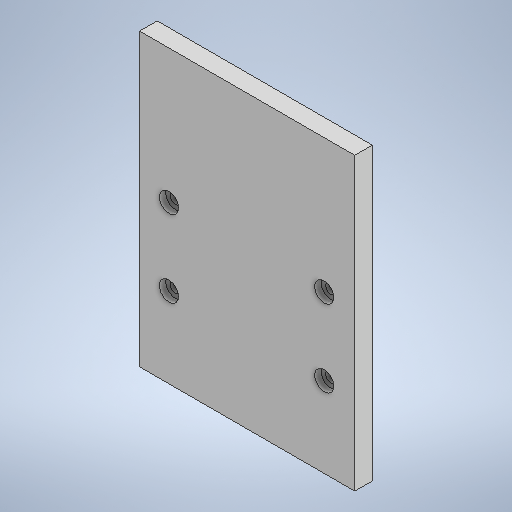
# Autodesk Inventor part: TES_ESP32-Case
Saved by Autodesk Inventor 2025 (Build 290162000, 162)
## iProperties
Created: 2025-08-28
Part Number: TES_ESP32-Case
Material: 常规
Document SubType Name: Modeling
Designer: user
Density: 1 g/cm^3
Appearance: 默认
Author: user
Autodesk Inventor part; units mm, degrees
ref_plane "YZ Plane" through (0, 0, 0) normal (1, 0, 0) x (0, 1, 0)
ref_plane "XZ Plane" through (0, 0, 0) normal (0, 1, 0) x (-1, 0, 0)
ref_plane "XY Plane" through (0, 0, 0) normal (0, 0, 1) x (1, 0, 0)
sketch "草图1" plane through (0, 0, 0) normal (0, 0, 1) x (1, 0, 0)
  line L0 (32.05, -44.65) -> (-32.05, -44.65)
  line L1 (-32.05, -44.65) -> (-32.05, 44.65)
  line L2 (-32.05, 44.65) -> (32.05, 44.65)
  line L3 (32.05, 44.65) -> (32.05, -44.65)
  line L4 (32.05, -44.65) -> (-32.05, 44.65) construction
  line L5 (-32.05, -44.65) -> (32.05, 44.65) construction
  line L6 (24.111, -19.563) -> (-24.389, -19.563) construction
  line L7 (-24.389, -19.563) -> (-24.389, 4.437) construction
  line L8 (-24.389, 4.437) -> (24.111, 4.437) construction
  line L9 (24.111, 4.437) -> (24.111, -19.563) construction
  line L10 (24.111, -19.563) -> (-24.389, 4.437) construction
  line L11 (-24.389, -19.563) -> (24.111, 4.437) construction
  circle A0 centre (-24.389, 4.437) radius 1.6
  circle A1 centre (-24.389, -19.563) radius 1.6
  circle A2 centre (24.111, 4.437) radius 1.6
  circle A3 centre (24.111, -19.563) radius 1.6
  line L12 (29.55, -43.15) -> (-4.45, -43.15)
  line L13 (-4.45, -43.15) -> (-4.45, -38.15)
  line L14 (-4.45, -38.15) -> (29.55, -38.15)
  line L15 (29.55, -38.15) -> (29.55, -43.15)
  line L16 (-19.55, -38.15) -> (-7.55, -38.15)
  line L17 (-7.55, -38.15) -> (-7.55, -33.65)
  line L18 (-7.55, -33.65) -> (-19.55, -33.65)
  line L19 (-19.55, -33.65) -> (-19.55, -38.15)
  line L20 (-20.05, -32.65) -> (-29.05, -32.65)
  line L21 (-29.05, -32.65) -> (-29.05, -28.15)
  line L22 (-29.05, -28.15) -> (-20.05, -28.15)
  line L23 (-20.05, -28.15) -> (-20.05, -32.65)
  line L24 (-12.05, 20.15) -> (-0.05, 20.15)
  line L25 (-0.05, 20.15) -> (-0.05, 24.65)
  line L26 (-0.05, 24.65) -> (-12.05, 24.65)
  line L27 (-12.05, 24.65) -> (-12.05, 20.15)
  point P0 (0, 0)
  point P1 (-0.139, -7.563)
  point P2 (-20.05, -30.4)
  dimension "d0" = 64.1
  dimension "d1" = 89.3
  dimension "d2" = 48.5
  dimension "d3" = 24
  dimension "d4" = 52.213
  dimension "d5" = 37.087
  dimension "d6" = 32.189
  dimension "d7" = 31.911
  dimension "d8" = 3.2
  dimension "d9" = 3.2
  dimension "d10" = 3.2
  dimension "d11" = 3.2
  dimension "d16" = 6.5
  dimension "d20" = 24.5
  dimension "d21" = 36.5
  dimension "d22" = 12.5
  dimension "d23" = 11
  dimension "d24" = 6.5
  dimension "d25" = 2.5
  dimension "d26" = 1.5
  dimension "d27" = 12
  dimension "d28" = 12
  dimension "d29" = 3
  dimension "d30" = 16.5
  dimension "d31" = 32
  dimension "d32" = 20
  dimension "d33" = 24.5
  dimension "d34" = 20
  constraints: 56 end point, 12 parallel, 6 horizontal, 6 perpendicular, 5 midpoint, 4 centre point, 4 coincident
  measures "d0" distance of L1.end L2.end
  measures "d1" distance of L0.end L1.end
  measures "d2" distance of L7.end L8.end
  measures "d3" distance of L6.end L7.end
  measures "d4" distance from line of L2 point (-0.139, -7.563)
  measures "d5" distance from line of point (-0.139, -7.563) L0
  measures "d6" distance from line of L3 point (-0.139, -7.563)
  measures "d7" distance from line of L1 point (-0.139, -7.563)
  measures "d8" diameter of A0
  measures "d9" diameter of A1
  measures "d10" diameter of A2
  measures "d11" diameter of A3
  measures "d16" distance between parallel lines of L0 L14
  measures "d20" distance between parallel lines of L1 L17
  measures "d21" distance between parallel lines of L3 L13
  measures "d22" distance between parallel lines of L1 L19
  measures "d23" distance between parallel lines of L0 L18
  measures "d24" distance between parallel lines of L0 L16
  measures "d25" distance between parallel lines of L3 L15
  measures "d26" distance between parallel lines of L0 L12
  measures "d27" distance between parallel lines of L0 L20
  measures "d28" distance from line of L1 point (-20.05, -30.4)
  measures "d29" distance between parallel lines of L1 L21
  measures "d30" distance between parallel lines of L0 L22
  measures "d31" distance between parallel lines of L1 L25
  measures "d32" distance between parallel lines of L1 L27
  measures "d33" distance between parallel lines of L2 L24
  measures "d34" distance between parallel lines of L2 L26
extrude "拉伸1" add sketch "草图1" along normal blind 2
sketch "草图2" plane through (0, 0, 2) normal (0, 0, 1) x (1, 0, 0)
  line L0 (-12.05, 20.15) -> (-12.05, 24.65) projected
  line L1 (-0.05, 24.65) -> (-0.05, 20.15) projected
  line L2 (-12.05, 24.65) -> (-0.05, 24.65)
  line L3 (-0.05, 24.65) -> (-0.05, 20.15)
  line L4 (-0.05, 20.15) -> (-12.05, 20.15)
  line L5 (-12.05, 20.15) -> (-12.05, 24.65)
  line L6 (-29.05, -32.65) -> (-29.05, -28.15) projected
  line L7 (-20.05, -32.65) -> (-29.05, -32.65) projected
  line L8 (-29.05, -28.15) -> (-20.05, -28.15)
  line L9 (-20.05, -28.15) -> (-20.05, -32.65)
  line L10 (-20.05, -32.65) -> (-29.05, -32.65)
  line L11 (-29.05, -32.65) -> (-29.05, -28.15)
  line L12 (-7.55, -33.65) -> (-7.55, -38.15) projected
  line L13 (-19.55, -33.65) -> (-7.55, -33.65)
  line L14 (-7.55, -33.65) -> (-7.55, -38.15)
  line L15 (-7.55, -38.15) -> (-19.55, -38.15)
  line L16 (-19.55, -38.15) -> (-19.55, -33.65)
  line L17 (-4.45, -43.15) -> (-4.45, -38.15) projected
  line L18 (29.55, -43.15) -> (-4.45, -43.15) projected
  line L19 (-4.45, -38.15) -> (29.55, -38.15)
  line L20 (29.55, -38.15) -> (29.55, -43.15)
  line L21 (29.55, -43.15) -> (-4.45, -43.15)
  line L22 (-4.45, -43.15) -> (-4.45, -38.15)
  line L23 (-32.05, -44.65) -> (32.05, -44.65) projected
  line L24 (32.05, -44.65) -> (-32.05, -44.65)
  line L25 (-32.05, -44.65) -> (-32.05, 44.65)
  line L26 (-32.05, 44.65) -> (32.05, 44.65)
  line L27 (32.05, 44.65) -> (32.05, -44.65)
  circle A0 centre (-24.389, 4.437) radius 1.6 projected
  circle A1 centre (-24.389, 4.437) radius 3
  circle A2 centre (-24.389, -19.563) radius 1.6 projected
  circle A3 centre (-24.389, -19.563) radius 3
  circle A4 centre (24.111, 4.437) radius 1.6 projected
  circle A5 centre (24.111, 4.437) radius 3
  circle A6 centre (24.111, -19.563) radius 3
  point P0 (0, 0)
  dimension "d37" = 6
  dimension "d38" = 6
  dimension "d39" = 6
  dimension "d40" = 6
  constraints: 40 end point, 10 parallel, 5 horizontal, 5 perpendicular, 4 centre point, 3 coincident
  measures "d37" diameter of A1
  measures "d38" diameter of A3
  measures "d39" diameter of A5
  measures "d40" diameter of A6
extrude "拉伸2" add sketch "草图2" along normal blind 1 contours L25 L26 L27 L23
sketch "草图3" plane through (0, 0, 3) normal (0, 0, 1) x (1, 0, 0)
  line L0 (-32.05, -44.65) -> (32.05, -44.65) projected
  line L1 (-32.05, 44.65) -> (-32.05, -44.65) projected
  line L2 (32.05, -44.65) -> (-32.05, -44.65)
  line L3 (-32.05, -44.65) -> (-32.05, 44.65)
  line L4 (-32.05, 44.65) -> (32.05, 44.65)
  line L5 (32.05, 44.65) -> (32.05, -44.65)
  circle A0 centre (-24.389, 4.437) radius 3 projected
  circle A1 centre (-24.389, 4.437) radius 3
  circle A2 centre (-24.389, -19.563) radius 3 projected
  circle A3 centre (-24.389, -19.563) radius 3
  circle A4 centre (24.111, -19.563) radius 3 projected
  circle A5 centre (24.111, -19.563) radius 3
  circle A6 centre (24.111, 4.437) radius 3 projected
  circle A7 centre (24.111, 4.437) radius 3
  point P0 (0, 0)
  constraints: 8 end point, 4 centre point, 4 coincident, 2 parallel, 1 horizontal, 1 perpendicular
extrude "拉伸3" add sketch "草图3" along normal blind 1
sketch "草图4" plane through (0, 0, 4) normal (0, 0, 1) x (1, 0, 0)
  line L0 (-32.05, 44.65) -> (-32.05, -44.65) projected
  line L1 (-32.05, -44.65) -> (32.05, -44.65) projected
  line L2 (-32.05, 44.65) -> (32.05, 44.65)
  line L3 (32.05, 44.65) -> (32.05, -44.65)
  line L4 (32.05, -44.65) -> (-32.05, -44.65)
  line L5 (-32.05, -44.65) -> (-32.05, 44.65)
  line L6 (33.628, 46.15) -> (-33.55, 46.15)
  line L7 (-33.55, 46.15) -> (-33.55, -44.65)
  line L8 (33.628, -44.65) -> (33.628, 46.15)
  line L9 (-33.55, -44.65) -> (33.628, -44.65)
  point P0 (0, 0)
  dimension "d45" = 1.5
  constraints: 16 end point, 3 parallel, 2 horizontal, 2 perpendicular, 1 other
  measures "d45" distance between parallel lines of L2 L6
extrude "拉伸4" add sketch "草图4" against normal blind 5.5 contours L0 L9 L7 L6 L8 L3 L2
